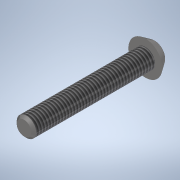
# Autodesk Inventor part: M8x50
Saved by Autodesk Inventor 2021 (Build 250183000, 183)
## iProperties
Created: 2024-04-18
Part Number: M8x50
Material: Ogólny
Document SubType Name: Modeling
Designer: Michal
Density: 1 g/cm^3
Appearance: Stainless - Brushed
Author: Michal
Autodesk Inventor part; units mm, degrees
ref_plane "YZ Plane" through (0, 0, 0) normal (1, 0, 0) x (0, 1, 0)
ref_plane "XZ Plane" through (0, 0, 0) normal (0, 1, 0) x (-1, 0, 0)
sketch "Sketch1" plane through (0, 0, 0) normal (0, 1, 0) x (-1, 0, 0)
  circle A0 centre (0, 0) radius 4
  dimension "d0" = 8
  constraints: 1 centre point, 1 coincident
  measures "d0" diameter of A0
extrude "Extrusion1" add sketch "Sketch1" along normal blind 50
chamfer "Chamfer1" distance 1 angle 45 1 edges at (4, 0, 0)
ref_plane "Work Plane1" through (0, 54.4, 0) normal (0, 1, 0) x (1, 0, 0)
thread "Thread1" size "M8x1.25" class "6g" standard "ANSI Metric M Profile" full length
sketch "Sketch5" plane through (0, 50, 0) normal (0, 1, 0) x (1, 0, 0)
  circle A0 centre (0, 0) radius 7
  dimension "d17" = 14
  constraints: 1 centre point, 1 coincident
  measures "d17" diameter of A0
sketch "Sketch6" plane through (0, 54.4, 0) normal (0, 1, 0) x (1, 0, 0)
  circle A0 centre (0, 0) radius 4
  dimension "d18" = 8
  constraints: 1 centre point, 1 coincident
  measures "d18" diameter of A0
loft "Loft2" add profiles "Sketch5", "Sketch6"
fillet "Fillet1" radius 2 1 edges at (-4, 54.4, 0)
sketch "Sketch7" plane through (0, 54.4, 0) normal (0, 1, 0) x (1, 0, 0)
  line L0 (2.8868, 0) -> (1.4434, -2.5)
  line L1 (1.4434, -2.5) -> (-1.4434, -2.5)
  line L2 (-1.4434, -2.5) -> (-2.8868, 0)
  line L3 (-2.8868, 0) -> (-1.4434, 2.5)
  line L4 (-1.4434, 2.5) -> (1.4434, 2.5)
  line L5 (1.4434, 2.5) -> (2.8868, 0)
  point P0 (0, 0)
  point P1 (0, 0)
  dimension "d24" = 5
  constraints: 12 end point, 1 coincident, 13 other
  measures "d24" distance between parallel lines of L1 L4
extrude "Extrusion3" cut sketch "Sketch7" against normal blind 5
body "Solid1"
